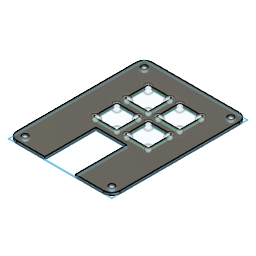
Mriduls_Hackpad_Keycaps_Cover (Autodesk Fusion 360 design; units mm, degrees)
part number: 2025-11-27-14-28-02-099
Autodesk Fusion 360 part; units mm, degrees
sketch "plate-2025-11-27T14_27_47.394Z" plane through (0, 0, 0) normal (0, 0, 1) x (1, 0, 0)
  line L0 (3.6469, -7.3061) -> (16.6469, -7.3061)
  line L1 (3.6469, -21.3061) -> (16.6469, -21.3061)
  line L2 (3.1469, -7.8061) -> (3.1469, -20.8061)
  line L3 (17.1469, -7.8061) -> (17.1469, -20.8061)
  arc A0 (3.6469, -7.3061) -> (3.1469, -7.8061) centre (3.6469, -7.8061) ccw
  arc A1 (17.1469, -7.8061) -> (16.6469, -7.3061) centre (16.6469, -7.8061) ccw
  arc A2 (3.1469, -20.8061) -> (3.6469, -21.3061) centre (3.6469, -20.8061) ccw
  arc A3 (16.6469, -21.3061) -> (17.1469, -20.8061) centre (16.6469, -20.8061) ccw
  line L4 (22.6969, -7.3061) -> (35.6969, -7.3061)
  line L5 (22.6969, -21.3061) -> (35.6969, -21.3061)
  line L6 (22.1969, -7.8061) -> (22.1969, -20.8061)
  line L7 (36.1969, -7.8061) -> (36.1969, -20.8061)
  arc A4 (22.6969, -7.3061) -> (22.1969, -7.8061) centre (22.6969, -7.8061) ccw
  arc A5 (36.1969, -7.8061) -> (35.6969, -7.3061) centre (35.6969, -7.8061) ccw
  arc A6 (22.1969, -20.8061) -> (22.6969, -21.3061) centre (22.6969, -20.8061) ccw
  arc A7 (35.6969, -21.3061) -> (36.1969, -20.8061) centre (35.6969, -20.8061) ccw
  line L8 (3.6469, -26.3561) -> (16.6469, -26.3561)
  line L9 (3.6469, -40.3561) -> (16.6469, -40.3561)
  line L10 (3.1469, -26.8561) -> (3.1469, -39.8561)
  line L11 (17.1469, -26.8561) -> (17.1469, -39.8561)
  arc A8 (3.6469, -26.3561) -> (3.1469, -26.8561) centre (3.6469, -26.8561) ccw
  arc A9 (17.1469, -26.8561) -> (16.6469, -26.3561) centre (16.6469, -26.8561) ccw
  arc A10 (3.1469, -39.8561) -> (3.6469, -40.3561) centre (3.6469, -39.8561) ccw
  arc A11 (16.6469, -40.3561) -> (17.1469, -39.8561) centre (16.6469, -39.8561) ccw
  line L12 (22.6969, -26.3561) -> (35.6969, -26.3561)
  line L13 (22.6969, -40.3561) -> (35.6969, -40.3561)
  line L14 (22.1969, -26.8561) -> (22.1969, -39.8561)
  line L15 (36.1969, -26.8561) -> (36.1969, -39.8561)
  arc A12 (22.6969, -26.3561) -> (22.1969, -26.8561) centre (22.6969, -26.8561) ccw
  arc A13 (36.1969, -26.8561) -> (35.6969, -26.3561) centre (35.6969, -26.8561) ccw
  arc A14 (22.1969, -39.8561) -> (22.6969, -40.3561) centre (22.6969, -39.8561) ccw
  arc A15 (35.6969, -40.3561) -> (36.1969, -39.8561) centre (35.6969, -39.8561) ccw
sketch "Sketch2" plane through (0, 0, 0) normal (0, 0, 1) x (1, 0, 0)
  line L0 (50.0469, -76.3561) -> (-12.4931, -76.3561)
  line L1 (-12.4931, -76.3561) -> (-12.4931, 5.8439)
  line L2 (-12.4931, 5.8439) -> (50.0469, 5.8439)
  line L3 (50.0469, 5.8439) -> (50.0469, -76.3561)
  line L4 (27.9369, -76.3561) -> (9.4369, -76.3561)
  line L5 (9.4369, -76.3561) -> (9.4369, -45.3561)
  line L6 (9.4369, -45.3561) -> (27.9369, -45.3561)
  line L7 (27.9369, -45.3561) -> (27.9369, -76.3561)
  circle A0 centre (45.0469, -71.3561) radius 1.7
  circle A1 centre (-7.4931, -71.3561) radius 1.7
  circle A2 centre (-7.4931, 0.8439) radius 1.7
  circle A3 centre (45.0469, 0.8439) radius 1.7
  line L8 (36.1897, -40.297) -> (22.134, -40.297)
  line L9 (22.134, -40.297) -> (22.134, -26.2413)
  line L10 (22.134, -26.2413) -> (36.1897, -26.2413)
  line L11 (36.1897, -26.2413) -> (36.1897, -40.297)
  line L12 (17.1676, -40.3908) -> (3.0182, -40.3908)
  line L13 (3.0182, -40.3908) -> (3.0182, -26.2413)
  line L14 (3.0182, -26.2413) -> (17.1676, -26.2413)
  line L15 (17.1676, -26.2413) -> (17.1676, -40.3908)
  line L16 (36.1897, -21.275) -> (22.134, -21.275)
  line L17 (22.134, -21.275) -> (22.134, -7.1256)
  line L18 (22.134, -7.1256) -> (36.1897, -7.1256)
  line L19 (36.1897, -7.1256) -> (36.1897, -21.275)
  line L20 (17.0739, -21.275) -> (3.0182, -21.275)
  line L21 (3.0182, -21.275) -> (3.0182, -7.1256)
  line L22 (3.0182, -7.1256) -> (17.0739, -7.1256)
  line L23 (17.0739, -7.1256) -> (17.0739, -21.275)
  dimension "d1" = 62.54
  dimension "d2" = 82.2
  dimension "d5" = 18.5
  dimension "d6" = 31
  dimension "d7" = 22.11
  dimension "d8" = 3.4
  dimension "d9" = 3.4
  dimension "d10" = 5
  dimension "d11" = 5
  dimension "d12" = 5
  dimension "d13" = 5
  dimension "d14" = 3.4
  dimension "d15" = 5
  dimension "d16" = 5
  dimension "d17" = 3.4
  dimension "d18" = 5
  dimension "d19" = 5
  constraint horizontal L0
  constraint vertical L1
  constraint horizontal L2
  constraint vertical L3
  constraint horizontal L4
  constraint vertical L5
  constraint horizontal L6
  constraint vertical L7
  constraint coincident L0 L4.start
  constraint horizontal L8
  constraint vertical L9
  constraint horizontal L10
  constraint vertical L11
  constraint horizontal L12
  constraint vertical L13
  constraint horizontal L14
  constraint vertical L15
  constraint horizontal L16
  constraint vertical L17
  constraint horizontal L18
  constraint vertical L19
  constraint horizontal L20
  constraint vertical L21
  constraint horizontal L22
  constraint vertical L23
  measures "d1" distance of L0.start L0.end
  measures "d2" distance of L0.start L2.end
  measures "d5" distance of L4.start L4.end
  measures "d6" distance of L4.start L6.end
  measures "d7" distance of L3 L7
  measures "d8" diameter of A0
  measures "d9" diameter of A1
  measures "d10" distance of L0 A0.centre
  measures "d11" distance of L3 A0.centre
  measures "d12" distance of L0 A1.centre
  measures "d13" distance of L1 A1.centre
  measures "d14" diameter of A2
  measures "d15" distance of L2 A2.centre
  measures "d16" distance of L1 A2.centre
  measures "d17" diameter of A3
  measures "d18" distance of L2 A3.centre
  measures "d19" distance of L3 A3.centre
extrude "Extrude1" add sketch "Sketch2" along normal blind 1.5 contours L0 L1 L2 L3 L5 L6 L7
fillet "Fillet1" radius 5 4 edges at (-12.4931, 5.8439, 0.75) (50.0469, 5.8439, 0.75) (50.0469, -76.3561, 0.75) (-12.4931, -76.3561, 0.75)
sketch "Sketch3" plane through (0, 0, 0) normal (0, 0, 1) x (1, 0, 0)
  line L0 (24.3243, -44.4459) -> (13.3243, -44.4459) construction
  line L1 (13.3243, -44.4459) -> (13.3243, -42.4459) construction
  line L2 (13.3243, -42.4459) -> (24.3243, -42.4459) construction
  line L3 (24.3243, -42.4459) -> (24.3243, -44.4459) construction
  dimension "d24" = 1
  text T0 "Mriduls Hackpad" font "Arial" height 1 align left top in box 11 x 2 at (24.3243, -44.4459) x (-1, 0) y (0, 1) spacing 1
extrude "Extrude2" add sketch "Sketch3" against normal blind 0.02 text T0
equation "d25 = 'Mriduls Hackpad'"
